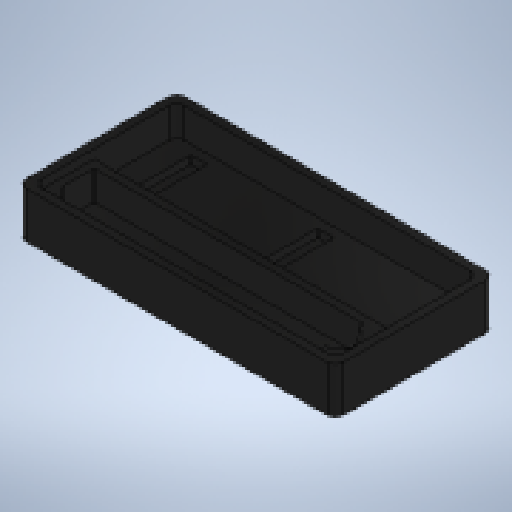
# Autodesk Inventor part: PinecilCaseBottom
Saved by Autodesk Inventor 2026 (Build 300175050, 175E)
## iProperties
Created: 2025-10-09
Part Number: PinecilCaseBottom
Material: Generic
Document SubType Name: Modeling
Designer: Nicholas M
Density: 1 g/cm^3
Appearance: Smooth - Black
Author: Nicholas M
Autodesk Inventor part; units mm, degrees
ref_plane "YZ Plane" through (0, 0, 0) normal (1, 0, 0) x (0, 1, 0)
ref_plane "XZ Plane" through (0, 0, 0) normal (0, 1, 0) x (-1, 0, 0)
ref_plane "XY Plane" through (0, 0, 0) normal (0, 0, 1) x (1, 0, 0)
sketch "Sketch1" plane through (0, 0, 0) normal (0, 1, 0) x (-1, 0, 0)
  line L0 (0, 0) -> (127, 0)
  line L1 (127, 0) -> (127, -63.5)
  line L2 (127, -63.5) -> (0, -63.5)
  line L3 (0, -63.5) -> (0, 0)
  line L4 (123.825, -60.325) -> (123.825, -3.175)
  line L5 (123.825, -3.175) -> (3.175, -3.175)
  line L6 (3.175, -3.175) -> (3.175, -60.325)
  line L7 (3.175, -60.325) -> (123.825, -60.325)
  dimension "d0" = 127
  dimension "d1" = 63.5
  dimension "d2" = 3.175
  constraints: 16 end point, 4 parallel, 2 perpendicular, 1 horizontal, 3 other
  measures "d0" distance of L1.end L2.end
  measures "d1" distance of L2.end L0.start
  measures "d2" distance between parallel lines of L1 L4
extrude "Extrusion1" add sketch "Sketch1" along normal blind 3.175 contours L0 L1 L2 L3 | L7 L6 L5 L4
extrude "Extrusion2" add sketch "Sketch1" along normal blind 18.415
fillet "Fillet1" radius 3.175 8 edges at (0, 9.2075, 0) (0, 9.2075, -63.5) (-127, 9.2075, -63.5) (-127, 9.2075, 0) (-123.825, 10.795, -3.175) (-3.175, 10.795, -3.175) (-123.825, 10.795, -60.325) (-3.175, 10.795, -60.325)
sketch "Sketch2" plane through (0, 3.175, 0) normal (0, 1, 0) x (1, 0, 0)
  line L0 (-120.65, 6.35) -> (-12.7, 6.35)
  line L1 (-12.7, 6.35) -> (-12.7, 24.13)
  line L2 (-12.7, 24.13) -> (-120.65, 24.13)
  line L3 (-120.65, 24.13) -> (-120.65, 6.35)
  line L4 (-3.175, 57.15) -> (-3.175, 6.35) projected
  line L5 (-6.35, 3.175) -> (-120.65, 3.175) projected
  line L6 (-24.892, 6.35) -> (-75.692, 6.35)
  line L7 (-75.692, 6.35) -> (-75.692, 5.588) construction
  line L8 (-75.692, 5.588) -> (-24.892, 5.588)
  line L9 (-24.892, 5.588) -> (-24.892, 6.35) construction
  line L10 (-24.892, 5.588) -> (-24.13, 6.35)
  line L11 (-123.825, 6.35) -> (-123.825, 57.15) projected
  line L12 (-75.692, 5.588) -> (-76.454, 6.35)
  line L13 (-123.825, 27.305) -> (-3.175, 27.305)
  arc A0 (-3.175, 57.15) -> (-6.35, 60.325) centre (-6.35, 57.15) ccw projected
  line L14 (-6.35, 60.325) -> (-120.65, 60.325) projected
  arc A1 (-120.65, 60.325) -> (-123.825, 57.15) centre (-120.65, 57.15) ccw projected
  line L15 (-123.825, 57.15) -> (-123.825, 6.35) projected
  arc A2 (-123.825, 6.35) -> (-120.65, 3.175) centre (-120.65, 6.35) ccw projected
  line L16 (-120.65, 3.175) -> (-6.35, 3.175) projected
  arc A3 (-6.35, 3.175) -> (-3.175, 6.35) centre (-6.35, 6.35) ccw projected
  line L17 (-3.175, 6.35) -> (-3.175, 57.15) projected
  point P0 (0, 0)
  dimension "d8" = 107.95
  dimension "d9" = 17.78
  dimension "d11" = 3.175
  dimension "d13" = 18.542
  dimension "d14" = 11.43
  dimension "d15" = 3.175
  dimension "d16" = 45
  dimension "d17" = 50.8
  dimension "d18" = 45
  dimension "d20" = 3.175
  constraints: 22 end point, 5 parallel, 5 point on line, 2 horizontal, 2 perpendicular
  measures "d8" distance of L2.end L1.end
  measures "d9" distance of L1.end L0.end
  measures "d11" distance between parallel lines of L5 L0
  measures "d13" distance between parallel lines of L2 L8
  measures "d14" distance of L0.end L10.end
  measures "d15" distance between parallel lines of L11 L3
  measures "d16" angle of L9 L10
  measures "d17" distance of L7.end L8.end
  measures "d18" angle of L7 L12
  measures "d20" distance between parallel lines of L2 L13
extrude "Extrusion3" add sketch "Sketch2" along normal blind 11.684 contours L4 A3 L5 A2 L11 L13
chamfer "Chamfer1" distance 5.08 angle 45 1 edges at (-120.65, 9.017, -6.35)
fillet "Fillet2" radius 0.7937 9 edges at (-76.454, 9.017, -6.35) (-75.692, 9.017, -5.588) (-24.892, 9.017, -5.588) (-24.13, 9.017, -6.35) (-12.7, 9.017, -6.35) (-12.7, 9.017, -24.13) (-120.65, 9.017, -24.13) (-120.65, 9.017, -11.43) (-115.57, 9.017, -6.35)
sketch "Sketch3" plane through (0, 14.859, 0) normal (0, 1, 0) x (1, 0, 0)
  line L0 (-12.7, 23.3363) -> (-12.7, 7.1438) projected
  circle A0 centre (-12.7, 15.24) radius 6.35
  line L1 (-6.35, 3.175) -> (-120.65, 3.175) projected
  arc A1 (-6.35, 3.175) -> (-3.175, 6.35) centre (-6.35, 6.35) ccw projected
  line L2 (-3.175, 27.305) -> (-3.175, 6.35) projected
  line L3 (-3.175, 27.305) -> (-123.825, 27.305) projected
  line L4 (-123.825, 6.35) -> (-123.825, 27.305) projected
  arc A2 (-123.825, 6.35) -> (-120.65, 3.175) centre (-120.65, 6.35) ccw projected
  arc A3 (-23.8012, 6.35) -> (-24.3625, 6.1175) centre (-23.8012, 5.5563) ccw projected
  line L5 (-24.3625, 6.1175) -> (-24.6595, 5.8205) projected
  arc A4 (-25.2208, 5.588) -> (-24.6595, 5.8205) centre (-25.2208, 6.3818) ccw projected
  line L6 (-25.2208, 5.588) -> (-75.3632, 5.588) projected
  arc A5 (-75.9245, 5.8205) -> (-75.3632, 5.588) centre (-75.3632, 6.3818) ccw projected
  line L7 (-75.9245, 5.8205) -> (-76.2215, 6.1175) projected
  arc A6 (-76.2215, 6.1175) -> (-76.7828, 6.35) centre (-76.7828, 5.5563) ccw projected
  line L8 (-76.7828, 6.35) -> (-115.2412, 6.35) projected
  arc A7 (-115.8025, 6.5825) -> (-115.2412, 6.35) centre (-115.2412, 7.1438) ccw projected
  line L9 (-120.4175, 11.1975) -> (-115.8025, 6.5825) projected
  arc A8 (-120.65, 11.7588) -> (-120.4175, 11.1975) centre (-119.8562, 11.7588) ccw projected
  line L10 (-120.65, 11.7588) -> (-120.65, 23.3363) projected
  arc A9 (-119.8562, 24.13) -> (-120.65, 23.3363) centre (-119.8562, 23.3363) ccw projected
  line L11 (-119.8562, 24.13) -> (-13.4937, 24.13) projected
  arc A10 (-12.7, 23.3363) -> (-13.4937, 24.13) centre (-13.4937, 23.3363) ccw projected
  line L12 (-12.7, 23.3363) -> (-12.7, 7.1438) projected
  arc A11 (-13.4937, 6.35) -> (-12.7, 7.1438) centre (-13.4937, 7.1438) ccw projected
  line L13 (-13.4937, 6.35) -> (-23.8012, 6.35) projected
  line L14 (-6.35, 5.5563) -> (-6.35, 25.4813)
  point P0 (0, 0)
  point P1 (-12.7, 21.59)
  point P2 (-12.7, 8.89)
  dimension "d27" = 3.175
  constraints: 2 end point, 1 centre point, 1 midpoint, 1 tangent, 1 vertical
  measures "d27" distance between parallel lines of L2 L14
revolve "Revolution1" cut sketch "Sketch3" angle 360 about axis through (-12.7, 14.859, -23.3363) along (0, 0, 1) picked at (-11.7816, 17.1471) contours A0 L0
fillet "Fillet3" radius 0.7937 1 edges at (-12.7, 8.509, -15.24)
sketch "Sketch4" plane through (0, 3.175, 0) normal (0, 1, 0) x (1, 0, 0)
  line L0 (-114.3, 31.115) -> (-107.95, 31.115)
  line L1 (-107.95, 31.115) -> (-107.95, 56.515)
  line L2 (-107.95, 56.515) -> (-114.3, 56.515)
  line L3 (-114.3, 56.515) -> (-114.3, 31.115)
  line L4 (-63.5, 31.115) -> (-57.15, 31.115)
  line L5 (-57.15, 31.115) -> (-57.15, 56.515)
  line L6 (-57.15, 56.515) -> (-63.5, 56.515)
  line L7 (-63.5, 56.515) -> (-63.5, 31.115)
  line L8 (-120.65, 60.325) -> (-6.35, 60.325) projected
  line L9 (-123.825, 6.35) -> (-123.825, 57.15) projected
  line L10 (-123.825, 27.305) -> (-3.175, 27.305) projected
  line L11 (-3.175, 27.305) -> (-3.175, 57.15) projected
  arc A0 (-3.175, 57.15) -> (-6.35, 60.325) centre (-6.35, 57.15) ccw projected
  line L12 (-6.35, 60.325) -> (-120.65, 60.325) projected
  arc A1 (-120.65, 60.325) -> (-123.825, 57.15) centre (-120.65, 57.15) ccw projected
  line L13 (-123.825, 57.15) -> (-123.825, 27.305) projected
  line L14 (-107.8865, 56.5785) -> (-107.8865, 31.0515)
  line L15 (-107.8865, 31.0515) -> (-114.3635, 31.0515)
  line L16 (-114.3635, 31.0515) -> (-114.3635, 56.5785)
  line L17 (-114.3635, 56.5785) -> (-107.8865, 56.5785)
  line L18 (-63.5635, 31.0515) -> (-57.0865, 31.0515)
  line L19 (-57.0865, 31.0515) -> (-57.0865, 56.5785)
  line L20 (-57.0865, 56.5785) -> (-63.5635, 56.5785)
  line L21 (-63.5635, 56.5785) -> (-63.5635, 31.0515)
  line L22 (-54.61, 59.055) -> (-54.61, 28.575)
  line L23 (-54.61, 28.575) -> (-66.04, 28.575)
  line L24 (-66.04, 28.575) -> (-66.04, 59.055)
  line L25 (-66.04, 59.055) -> (-54.61, 59.055)
  line L26 (-105.41, 59.055) -> (-105.41, 28.575)
  line L27 (-105.41, 28.575) -> (-116.84, 28.575)
  line L28 (-116.84, 28.575) -> (-116.84, 59.055)
  line L29 (-116.84, 59.055) -> (-105.41, 59.055)
  point P0 (0, 0)
  point P1 (-111.125, 56.515)
  point P2 (-60.325, 56.515)
  dimension "d30" = 6.35
  dimension "d31" = 25.4
  dimension "d32" = 6.35
  dimension "d33" = 25.4
  dimension "d34" = 50.8
  dimension "d35" = 3.81
  dimension "d36" = 12.7
  dimension "d40" = 0.0635
  dimension "d41" = 0.0635
  dimension "d42" = 2.54
  dimension "d43" = 2.54
  constraints: 48 end point, 12 parallel, 6 perpendicular, 2 horizontal, 2 midpoint, 1 horizontal alignment, 12 other
  measures "d30" distance of L2.end L1.end
  measures "d31" distance of L1.end L0.end
  measures "d32" distance of L6.end L5.end
  measures "d33" distance of L5.end L4.end
  measures "d34" distance of point (-111.125, 56.515) point (-60.325, 56.515)
  measures "d35" distance between parallel lines of L8 L6
  measures "d36" distance from line of L9 point (-111.125, 56.515)
  measures "d40" distance between parallel lines of L1 L14
  measures "d41" distance between parallel lines of L7 L21
  measures "d42" distance between parallel lines of L5 L22
  measures "d43" distance between parallel lines of L1 L26
extrude "Extrusion4" add sketch "Sketch4" along normal blind 3.175 contours L22 L23 L24 L25 | L26 L27 L28 L29
fillet "Fillet4" radius 0.7937 16 edges at (-63.5635, 4.7625, -31.0515) (-57.0865, 4.7625, -31.0515) (-57.0865, 4.7625, -56.5785) (-63.5635, 4.7625, -56.5785) (-107.8865, 4.7625, -56.5785) (-114.3635, 4.7625, -56.5785) (-114.3635, 4.7625, -31.0515) (-107.8865, 4.7625, -31.0515) (-54.61, 4.7625, -28.575) (-66.04, 4.7625, -28.575) (-66.04, 4.7625, -59.055) (-54.61, 4.7625, -59.055) (-105.41, 4.7625, -59.055) (-116.84, 4.7625, -59.055) (-116.84, 4.7625, -28.575) (-105.41, 4.7625, -28.575)
body "Solid1"
